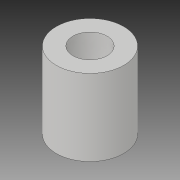
# Autodesk Inventor part: am-1307
Saved by Autodesk Inventor 2018 (Build 220112000, 112)
## iProperties
Category: Chassis Kit 2
Company: Autodesk Inc.
Created: 2017-12-13
Part Number: am-1307
Material: Generic
Document SubType Name: Modeling
Designer: Autodesk Inc.
Density: 1 g/cm^3
Appearance: Default
Catalog Web Link: http://www.andymark.com/product-p/am-1307.htm
Vendor: AndyMark Inc.
Author: Autodesk Inc.
Keywords: Drive Base Kit
Autodesk Inventor part; units mm, degrees
ref_plane "YZ Plane" through (0, 0, 0) normal (1, 0, 0) x (0, 1, 0)
ref_plane "XZ Plane" through (0, 0, 0) normal (0, 1, 0) x (-1, 0, 0)
ref_plane "XY Plane" through (0, 0, 0) normal (0, 0, 1) x (1, 0, 0)
sketch "Sketch1" plane through (0, 0, 0) normal (0, 1, 0) x (-1, 0, 0)
  circle A0 centre (0, 0) radius 9.525
  circle A1 centre (0, 0) radius 4.826
  dimension "d0" = 19.05
  dimension "d3" = 9.652
  constraints: 2 centre point, 2 coincident
  measures "d0" diameter of A0
  measures "d3" diameter of A1
extrude "Extrusion1" add sketch "Sketch1" against normal blind 21.59
body "Solid1"
